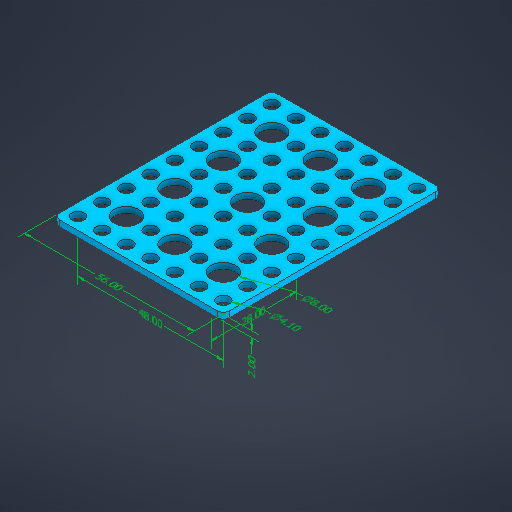
# Autodesk Inventor part: Plate 7x9
Saved by Autodesk Inventor 2026.1 (Build 301233020, 233B)
## iProperties
Created: 2025-10-11
Part Number: Plate 7x9
Material: Generic
Document SubType Name: Modeling
Designer: Asus
Density: 1 g/cm^3
Appearance: Default
Author: Asus
Autodesk Inventor part; units mm, degrees
ref_plane "YZ Plane" through (0, 0, 0) normal (1, 0, 0) x (0, 1, 0)
ref_plane "XZ Plane" through (0, 0, 0) normal (0, 1, 0) x (-1, 0, 0)
ref_plane "XY Plane" through (0, 0, 0) normal (0, 0, 1) x (1, 0, 0)
sketch "Sketch1" plane through (0, 0, 0) normal (0, 1, 0) x (-1, 0, 0)
  line L0 (-2, 0) -> (-54, 0)
  line L1 (-56, -2) -> (-56, -70)
  line L2 (-54, -72) -> (-2, -72)
  line L3 (0, -70) -> (0, -2)
  arc A0 (-2, -72) -> (0, -70) centre (-2, -70) ccw
  arc A1 (-56, -70) -> (-54, -72) centre (-54, -70) ccw
  arc A2 (-54, 0) -> (-56, -2) centre (-54, -2) ccw
  arc A3 (0, -2) -> (-2, 0) centre (-2, -2) ccw
  circle A4 centre (-4, -68) radius 2.05
  circle A5 centre (-12, -68) radius 2.05
  circle A6 centre (-20, -68) radius 2.05
  circle A7 centre (-28, -68) radius 2.05
  circle A8 centre (-36, -68) radius 2.05
  circle A9 centre (-44, -68) radius 2.05
  circle A10 centre (-52, -68) radius 2.05
  circle A11 centre (-4, -60) radius 2.05
  circle A12 centre (-12, -60) radius 2.05
  circle A13 centre (-20, -60) radius 2.05
  circle A14 centre (-28, -60) radius 2.05
  circle A15 centre (-36, -60) radius 2.05
  circle A16 centre (-44, -60) radius 2.05
  circle A17 centre (-52, -60) radius 2.05
  circle A18 centre (-4, -52) radius 2.05
  circle A19 centre (-12, -52) radius 2.05
  circle A20 centre (-20, -52) radius 2.05
  circle A21 centre (-28, -52) radius 2.05
  circle A22 centre (-36, -52) radius 2.05
  circle A23 centre (-44, -52) radius 2.05
  circle A24 centre (-52, -52) radius 2.05
  circle A25 centre (-4, -44) radius 2.05
  circle A26 centre (-12, -44) radius 2.05
  circle A27 centre (-20, -44) radius 2.05
  circle A28 centre (-28, -44) radius 2.05
  circle A29 centre (-36, -44) radius 2.05
  circle A30 centre (-44, -44) radius 2.05
  circle A31 centre (-52, -44) radius 2.05
  circle A32 centre (-4, -36) radius 2.05
  circle A33 centre (-12, -36) radius 2.05
  circle A34 centre (-20, -36) radius 2.05
  circle A35 centre (-28, -36) radius 2.05
  circle A36 centre (-36, -36) radius 2.05
  circle A37 centre (-44, -36) radius 2.05
  circle A38 centre (-52, -36) radius 2.05
  circle A39 centre (-4, -28) radius 2.05
  circle A40 centre (-12, -28) radius 2.05
  circle A41 centre (-20, -28) radius 2.05
  circle A42 centre (-28, -28) radius 2.05
  circle A43 centre (-36, -28) radius 2.05
  circle A44 centre (-44, -28) radius 2.05
  circle A45 centre (-52, -28) radius 2.05
  circle A46 centre (-4, -20) radius 2.05
  circle A47 centre (-12, -20) radius 2.05
  circle A48 centre (-20, -20) radius 2.05
  circle A49 centre (-28, -20) radius 2.05
  circle A50 centre (-36, -20) radius 2.05
  circle A51 centre (-44, -20) radius 2.05
  circle A52 centre (-52, -20) radius 2.05
  circle A53 centre (-4, -12) radius 2.05
  circle A54 centre (-12, -12) radius 2.05
  circle A55 centre (-20, -12) radius 2.05
  circle A56 centre (-28, -12) radius 2.05
  circle A57 centre (-36, -12) radius 2.05
  circle A58 centre (-44, -12) radius 2.05
  circle A59 centre (-52, -12) radius 2.05
  circle A60 centre (-4, -4) radius 2.05
  circle A61 centre (-12, -4) radius 2.05
  circle A62 centre (-20, -4) radius 2.05
  circle A63 centre (-28, -4) radius 2.05
  circle A64 centre (-36, -4) radius 2.05
  circle A65 centre (-44, -4) radius 2.05
  circle A66 centre (-52, -4) radius 2.05
  circle A67 centre (-44, -12) radius 4
  circle A68 centre (-12, -12) radius 4
  circle A69 centre (-28, -12) radius 4
  circle A70 centre (-28, -36) radius 4
  circle A71 centre (-44, -28) radius 4
  circle A72 centre (-12, -28) radius 4
  circle A73 centre (-12, -44) radius 4
  circle A74 centre (-44, -44) radius 4
  circle A75 centre (-44, -60) radius 4
  circle A76 centre (-28, -60) radius 4
  circle A77 centre (-12, -60) radius 4
  point P0 (0, 0)
  point P1 (-56, -72)
  point P2 (-56, 0)
  point P3 (0, -72)
  dimension "d0" = 56
  dimension "d1" = 72
  dimension "d2" = 2
  dimension "d3" = 4.1
  dimension "d5" = 4
  dimension "d8" = 8
  dimension "d11" = 8
  dimension "d14" = 8
  dimension "d15" = 8
  dimension "d16" = 8
  dimension "d17" = 8
  dimension "d18" = 8
  dimension "d19" = 8
  dimension "d20" = 8
  dimension "d21" = 8
  dimension "d22" = 8
  dimension "d23" = 8
  dimension "d24" = 8
  constraints: 78 centre point, 11 coincident, 8 end point, 8 point on circle, 8 point on line, 8 tangent, 3 equal radius, 2 horizontal, 2 parallel, 1 perpendicular, 1 vertical, 124 other
  measures "d0" distance of point (0, -72) point (-56, -72)
  measures "d1" distance of point (-56, -72) point (-56, 0)
  measures "d2" radius of A0
  measures "d3" diameter of A4
  measures "d5" distance from line of L3 A4.centre
  measures "d8" distance of A4.centre A5.centre
  measures "d11" distance of A4.centre A11.centre
  measures "d14" diameter of A67
  measures "d15" diameter of A68
  measures "d16" diameter of A69
  measures "d17" diameter of A70
  measures "d18" diameter of A71
  measures "d19" diameter of A72
  measures "d20" diameter of A73
  measures "d21" diameter of A74
  measures "d22" diameter of A75
  measures "d23" diameter of A76
  measures "d24" diameter of A77
extrude "Extrusion1" add sketch "Sketch1" along normal blind 2 contours A3 L3 A0 L2 A1 L1 A2 L0
body "Solid1"
